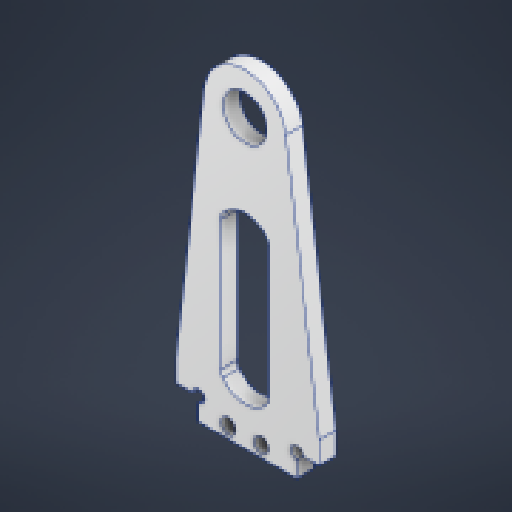
# Autodesk Inventor part: Leg_joint_slider_frame
Saved by Autodesk Inventor 2024 (Build 280153000, 153)
## iProperties
Created: 2024-01-23
Part Number: Leg_joint_slider_frame
Material: 알루미늄 6061
Document SubType Name: Modeling
Designer: ASUS
Density: 2.7 g/cm^3
Appearance: 알루미늄 - 평지
Mass: 6.96324 g
Surface Area: 24.9721 cm^2
Volume: 2.57898 cm^3
Author: ASUS
Autodesk Inventor part; units mm, degrees
ref_plane "YZ Plane" through (0, 0, 0) normal (1, 0, 0) x (0, 1, 0)
ref_plane "XZ Plane" through (0, 0, 0) normal (0, 1, 0) x (-1, 0, 0)
ref_plane "XY Plane" through (0, 0, 0) normal (0, 0, 1) x (1, 0, 0)
sketch "스케치1" plane through (0, 0, 0) normal (0, 0, 1) x (1, 0, 0)
  circle A0 centre (3, 0) radius 3 projected
  line L0 (7.4, -0.9434) -> (7.4, 0.9434) projected
  arc A1 (7.4, 0.9434) -> (-1.4, 0.9434) centre (3, 0) ccw projected
  line L1 (-1.4, 0.9434) -> (-1.4, -0.9434) projected
  arc A2 (-1.4, -0.9434) -> (7.4, -0.9434) centre (3, 0) ccw projected
  circle A3 centre (3, 20) radius 2.75 projected
  line L2 (3, 20) -> (3, 0)
  line L3 (3, 20) -> (3, 40)
  circle A4 centre (3, 40) radius 2.75
  circle A5 centre (3, 40) radius 7.5
  circle A6 centre (3, 0) radius 12.5
  line L4 (16.7123, -8.8378) -> (8.966, 52.6461)
  line L5 (-2.8681, 53.4235) -> (-11.5752, -15.6873)
  point P0 (0, 0)
  point P1 (10.4412, 40.9375)
  point P2 (-4.4412, 40.9375)
  point P3 (-9.402, 1.5625)
  point P4 (15.402, 1.5625)
  dimension "d2" = 360
  dimension "d4" = 5.5
  dimension "d5" = 15
  dimension "d6" = 25
  constraints: 8 end point, 5 coincident, 4 tangent, 3 centre point, 1 horizontal alignment, 1 vertical, 5 other
  measures "d4" diameter of A4
  measures "d5" diameter of A5
  measures "d6" diameter of A6
extrude "돌출1" add sketch "스케치1" along normal blind 3 contours A3 L3 A5 L4 A6 L2 | A3 L2 A6 L5 A5 L3 | A5 | A6
sketch "스케치2" plane through (0, 0, 3) normal (0, 0, 1) x (1, 0, 0)
  line L0 (-4.4412, 40.9375) -> (-9.402, 1.5625) projected
  arc A0 (-9.402, 1.5625) -> (15.402, 1.5625) centre (3, 0) ccw projected
  line L1 (15.402, 1.5625) -> (10.4412, 40.9375) projected
  arc A1 (10.4412, 40.9375) -> (-4.4412, 40.9375) centre (3, 40) ccw projected
  circle A2 centre (3, 40) radius 2.75 projected
  circle A3 centre (3, 20) radius 2.75 projected
  arc A4 (7.4, 0.9434) -> (-1.4, 0.9434) centre (3, 0) ccw projected
  line L2 (7.4, 0.9434) -> (7.4, -0.9434) projected
  arc A5 (-1.4, -0.9434) -> (7.4, -0.9434) centre (3, 0) ccw projected
  line L3 (-1.4, -0.9434) -> (-1.4, 0.9434) projected
  line L4 (-1.4, 14.3273) -> (-1.4, 9.5775) projected
  arc A6 (7.4, 14.3273) -> (-1.4, 14.3273) centre (3, 11.9524) ccw projected
  line L5 (7.4, 9.5775) -> (7.4, 14.3273) projected
  arc A7 (-1.4, 9.5775) -> (7.4, 9.5775) centre (3, 11.9524) ccw projected
  circle A8 centre (3, 11.9524) radius 6 projected
  line L6 (-1.4, 14.3273) -> (-1.4, -0.9434)
  line L7 (7.4, 14.3273) -> (7.4, -0.9434)
  point P0 (0, 0)
  point P1 (-1.4, 0.9434)
  point P2 (7.4, 0.9434)
  constraints: 4 end point, 1 parallel, 1 vertical
extrude "돌출2" cut sketch "스케치2" against normal up to surface (3 mm away) contours L6 A7 L7 A8 | A8 L7 A4 L6 | L4 A6 L5 A7
sketch "스케치3" plane through (0, 0, 0) normal (0, 0, -1) x (-1, 0, 0)
  circle A0 centre (-3, 40) radius 3.7 projected
  point P0 (0, 0)
extrude "돌출3" cut sketch "스케치3" against normal through all
sketch "스케치4" plane through (0, 0, 3) normal (0, 0, 1) x (1, 0, 0)
  circle A0 centre (3, 40) radius 4 projected
  circle A1 centre (3, 40) radius 3.7 projected
  line L0 (-1.4, -0.9434) -> (-1.4, 14.3273) projected
  arc A2 (7.4, 14.3273) -> (-1.4, 14.3273) centre (3, 11.9524) ccw projected
  line L1 (7.4, 14.3273) -> (7.4, -0.9434) projected
  arc A3 (-1.4, -0.9434) -> (7.4, -0.9434) centre (3, 0) ccw projected
  circle A4 centre (3, 20) radius 2.75 projected
  line L2 (-4.4412, 40.9375) -> (-9.402, 1.5625) projected
  arc A5 (-9.402, 1.5625) -> (15.402, 1.5625) centre (3, 0) ccw projected
  line L3 (15.402, 1.5625) -> (10.4412, 40.9375) projected
  arc A6 (10.4412, 40.9375) -> (-4.4412, 40.9375) centre (3, 40) ccw projected
  point P0 (0, 0)
extrude "돌출4" cut sketch "스케치4" against normal through all contours A0 | A1
sketch "스케치5" plane through (0, 0, 3) normal (0, 0, 1) x (1, 0, 0)
  circle A0 centre (3, 40) radius 4 projected
  line L0 (-1.4, -0.9434) -> (-1.4, 14.3273) projected
  arc A1 (7.4, 14.3273) -> (-1.4, 14.3273) centre (3, 11.9524) ccw projected
  line L1 (7.4, 14.3273) -> (7.4, -0.9434) projected
  arc A2 (-1.4, -0.9434) -> (7.4, -0.9434) centre (3, 0) ccw projected
  circle A3 centre (3, 20) radius 2.75 projected
  line L2 (-4.4412, 40.9375) -> (-9.402, 1.5625) projected
  arc A4 (-9.402, 1.5625) -> (15.402, 1.5625) centre (3, 0) ccw projected
  line L3 (15.402, 1.5625) -> (10.4412, 40.9375) projected
  arc A5 (10.4412, 40.9375) -> (-4.4412, 40.9375) centre (3, 40) ccw projected
  point P0 (0, 0)
extrude "돌출5" add sketch "스케치5" against normal up to surface (3 mm away) contours A3
sketch "스케치6" plane through (0, 0, 3) normal (0, 0, 1) x (1, 0, 0)
  circle A0 centre (3, 40) radius 4 projected
  line L0 (-1.4, -0.9434) -> (-1.4, 14.3273) projected
  arc A1 (7.4, 14.3273) -> (-1.4, 14.3273) centre (3, 11.9524) ccw projected
  line L1 (7.4, 14.3273) -> (7.4, -0.9434) projected
  arc A2 (-1.4, -0.9434) -> (7.4, -0.9434) centre (3, 0) ccw projected
  line L2 (-4.4412, 40.9375) -> (-9.402, 1.5625) projected
  arc A3 (-9.402, 1.5625) -> (15.402, 1.5625) centre (3, 0) ccw projected
  line L3 (15.402, 1.5625) -> (10.4412, 40.9375) projected
  arc A4 (10.4412, 40.9375) -> (-4.4412, 40.9375) centre (3, 40) ccw projected
  line L4 (-6.4255, 1.1875) -> (-1.4647, 40.5625)
  arc A5 (7.4647, 40.5625) -> (-1.4647, 40.5625) centre (3, 40) ccw
  line L5 (7.4647, 40.5625) -> (12.4255, 1.1875)
  arc A6 (-6.4255, 1.1875) -> (12.4255, 1.1875) centre (3, 0) ccw
  circle A7 centre (3, 40) radius 7
  circle A8 centre (3, 11.9524) radius 8.0059
  point P0 (0, 0)
  point P1 (-4.9432, 12.9531)
  point P2 (10.9432, 12.9531)
  point P3 (8.1349, 35.2427)
  point P4 (-2.1349, 35.2427)
  dimension "d17" = 3
  dimension "d18" = 3
  constraints: 4 centre point, 4 end point, 4 point on circle, 1 coincident, 1 tangent, 3 other
  measures "d17" distance between parallel lines of L2 L4
  measures "d18" radial gap between concentric circles of A0 A7
extrude "돌출6" cut sketch "스케치6" against normal through all contours L4 A7 L5 A8
fillet "모깎기1" radius 2 4 edges at (-2.1349, 35.2427, 1.5) (8.1349, 35.2427, 1.5) (-4.9432, 12.9531, 1.5) (10.9432, 12.9531, 1.5)
sketch "스케치8" plane through (0, 0, 3) normal (0, 0, 1) x (1, 0, 0)
  arc A0 (0.2302, 33.5713) -> (5.7698, 33.5713) centre (3, 40) ccw projected
  arc A1 (0.2302, 33.5713) -> (-2.5454, 31.9845) centre (-0.5611, 31.7345) ccw projected
  line L0 (-2.5454, 31.9845) -> (-3.9428, 20.8933) projected
  arc A2 (-3.9428, 20.8933) -> (-0.9674, 18.9062) centre (-1.9585, 20.6433) ccw projected
  arc A3 (6.9674, 18.9062) -> (-0.9674, 18.9062) centre (3, 11.9524) ccw projected
  arc A4 (6.9674, 18.9062) -> (9.9428, 20.8933) centre (7.9585, 20.6433) ccw projected
  line L1 (9.9428, 20.8933) -> (8.5454, 31.9845) projected
  arc A5 (8.5454, 31.9845) -> (5.7698, 33.5713) centre (6.5611, 31.7345) ccw projected
  circle A6 centre (3, 40) radius 4 projected
  line L2 (-1.4, 14.3273) -> (-1.4, -0.9434) projected
  arc A7 (-1.4, -0.9434) -> (7.4, -0.9434) centre (3, 0) ccw projected
  line L3 (7.4, -0.9434) -> (7.4, 14.3273) projected
  arc A8 (7.4, 14.3273) -> (-1.4, 14.3273) centre (3, 11.9524) ccw projected
  line L4 (-4.4412, 40.9375) -> (-9.402, 1.5625) projected
  arc A9 (10.4412, 40.9375) -> (-4.4412, 40.9375) centre (3, 40) ccw projected
  line L5 (15.402, 1.5625) -> (10.4412, 40.9375) projected
  arc A10 (-9.402, 1.5625) -> (15.402, 1.5625) centre (3, 0) ccw projected
  arc A11 (-1.4, 9.3409) -> (7.4, 9.3409) centre (3, 11.7157) ccw projected
  arc A12 (7.4, 14.0906) -> (-1.4, 14.0906) centre (3, 11.7157) ccw projected
  point P0 (0, 0)
extrude "돌출8" add sketch "스케치8" against normal up to surface (3 mm away) contours A8 L3 A12 L2
sketch "스케치9" plane through (0, 0, 0) normal (0, 0, -1) x (-1, 0, 0)
  line L0 (10.45, -12) -> (-15.45, -12)
  line L1 (10.45, -12) -> (10.45, -8)
  line L2 (-15.45, -8) -> (10.45, -8)
  line L3 (-15.45, -12) -> (-15.45, -8)
  arc A0 (-5.7698, 33.5713) -> (-0.2302, 33.5713) centre (-3, 40) ccw projected
  arc A1 (2.5454, 31.9845) -> (-0.2302, 33.5713) centre (0.5611, 31.7345) ccw projected
  line L4 (2.5454, 31.9845) -> (3.9428, 20.8933) projected
  arc A2 (0.9674, 18.9062) -> (3.9428, 20.8933) centre (1.9585, 20.6433) ccw projected
  arc A3 (0.9674, 18.9062) -> (-6.9674, 18.9062) centre (-3, 11.9524) ccw projected
  arc A4 (-9.9428, 20.8933) -> (-6.9674, 18.9062) centre (-7.9585, 20.6433) ccw projected
  line L5 (-9.9428, 20.8933) -> (-8.5454, 31.9845) projected
  arc A5 (-5.7698, 33.5713) -> (-8.5454, 31.9845) centre (-6.5611, 31.7345) ccw projected
  circle A6 centre (-3, 40) radius 4 projected
  line L6 (1.4, 14.0906) -> (1.4, -0.9434) projected
  arc A7 (-7.4, -0.9434) -> (1.4, -0.9434) centre (-3, 0) ccw projected
  line L7 (-7.4, -0.9434) -> (-7.4, 14.0906) projected
  arc A8 (1.4, 14.0906) -> (-7.4, 14.0906) centre (-3, 11.7157) ccw projected
  line L8 (4.4412, 40.9375) -> (9.402, 1.5625) projected
  arc A9 (4.4412, 40.9375) -> (-10.4412, 40.9375) centre (-3, 40) ccw projected
  line L9 (-15.402, 1.5625) -> (-10.4412, 40.9375) projected
  arc A10 (-15.402, 1.5625) -> (9.402, 1.5625) centre (-3, 0) ccw projected
  circle A11 centre (-3, 0) radius 12.5
  line L10 (-3, 0) -> (-15.5, 0)
  line L11 (-15.5, 0) -> (9.5, 0)
  line L12 (9.5, 0) -> (-15.5, 0)
  line L13 (-15.5, 0) -> (-15.5, -12)
  line L14 (-15.5, -12) -> (9.5, -12)
  line L15 (9.5, -12) -> (9.5, 0)
  point P0 (0, 0)
  point P1 (-6.5, -12)
  point P2 (0.5, -12)
  constraints: 20 end point, 3 equal length, 3 horizontal, 2 point on circle, 2 vertical, 1 centre point, 1 coincident, 1 perpendicular, 4 other
extrude "돌출9" add sketch "스케치9" against normal up to surface (3 mm away) contours L0 A10 L2 L15 | L2 A10 L15 | L0 L3 L2 A10 | L14 L13 A10 L2 L3
sketch "스케치10" plane through (0, 0, 0) normal (0, 0, -1) x (-1, 0, 0)
  arc A0 (-5.7698, 33.5713) -> (-0.2302, 33.5713) centre (-3, 40) ccw projected
  arc A1 (2.5454, 31.9845) -> (-0.2302, 33.5713) centre (0.5611, 31.7345) ccw projected
  line L0 (2.5454, 31.9845) -> (3.9428, 20.8933) projected
  arc A2 (0.9674, 18.9062) -> (3.9428, 20.8933) centre (1.9585, 20.6433) ccw projected
  arc A3 (0.9674, 18.9062) -> (-6.9674, 18.9062) centre (-3, 11.9524) ccw projected
  arc A4 (-9.9428, 20.8933) -> (-6.9674, 18.9062) centre (-7.9585, 20.6433) ccw projected
  line L1 (-9.9428, 20.8933) -> (-8.5454, 31.9845) projected
  arc A5 (-5.7698, 33.5713) -> (-8.5454, 31.9845) centre (-6.5611, 31.7345) ccw projected
  circle A6 centre (-3, 40) radius 4 projected
  line L2 (1.4, 14.0906) -> (1.4, -0.9434) projected
  arc A7 (-7.4, -0.9434) -> (1.4, -0.9434) centre (-3, 0) ccw projected
  line L3 (-7.4, -0.9434) -> (-7.4, 14.0906) projected
  arc A8 (1.4, 14.0906) -> (-7.4, 14.0906) centre (-3, 11.7157) ccw projected
  line L4 (4.4412, 40.9375) -> (9.402, 1.5625) projected
  arc A9 (4.4412, 40.9375) -> (-10.4412, 40.9375) centre (-3, 40) ccw projected
  line L5 (-15.402, 1.5625) -> (-10.4412, 40.9375) projected
  arc A10 (-15.402, 1.5625) -> (-15.5, 0) centre (-3, 0) ccw projected
  line L6 (-15.5, 0) -> (-15.5, -12) projected
  line L7 (-15.5, -12) -> (-6.5, -12) projected
  arc A11 (-6.5, -12) -> (0.5, -12) centre (-3, 0) ccw projected
  line L8 (0.5, -12) -> (9.5, -12) projected
  line L9 (9.5, -12) -> (9.5, 0) projected
  arc A12 (9.5, 0) -> (9.402, 1.5625) centre (-3, 0) ccw projected
  line L10 (9.5, -12) -> (-15.5, -12)
  point P0 (0, 0)
  constraints: 2 end point, 1 horizontal
extrude "돌출10" cut sketch "스케치10" against normal through all contours A11 L10
sketch "스케치11" plane through (0, 0, 0) normal (0, 0, -1) x (-1, 0, 0)
  line L0 (-8.5, -12) -> (3.5, -12)
  line L1 (-8.5, -8) -> (-8.5, -12)
  line L2 (3.5, -8) -> (-8.5, -8)
  line L3 (3.5, -12) -> (3.5, -8)
  line L4 (3.5, -10) -> (0.5, -10)
  line L5 (3.5, -10) -> (6.5, -10) construction
  line L6 (-8.5, -10) -> (-5.5, -10)
  line L7 (-8.5, -10) -> (-5.5, -10) construction
  circle A0 centre (0.5, -10) radius 1.35
  circle A1 centre (-5.5, -10) radius 1.35
  line L8 (-15.5, -12) -> (9.5, -12) projected
  line L9 (9.5, -12) -> (9.5, 0) projected
  arc A2 (9.5, 0) -> (9.402, 1.5625) centre (-3, 0) ccw projected
  line L10 (4.4412, 40.9375) -> (9.402, 1.5625) projected
  arc A3 (4.4412, 40.9375) -> (-10.4412, 40.9375) centre (-3, 40) ccw projected
  line L11 (-15.402, 1.5625) -> (-10.4412, 40.9375) projected
  arc A4 (-15.402, 1.5625) -> (-15.5, 0) centre (-3, 0) ccw projected
  line L12 (-15.5, 0) -> (-15.5, -12) projected
  line L13 (1.4, 14.0906) -> (1.4, -0.9434) projected
  arc A5 (-7.4, -0.9434) -> (1.4, -0.9434) centre (-3, 0) ccw projected
  line L14 (-7.4, -0.9434) -> (-7.4, 14.0906) projected
  arc A6 (1.4, 14.0906) -> (-7.4, 14.0906) centre (-3, 11.7157) ccw projected
  circle A7 centre (-3, 40) radius 4 projected
  arc A8 (-5.7698, 33.5713) -> (-0.2302, 33.5713) centre (-3, 40) ccw projected
  arc A9 (2.5454, 31.9845) -> (-0.2302, 33.5713) centre (0.5611, 31.7345) ccw projected
  line L15 (2.5454, 31.9845) -> (3.9428, 20.8933) projected
  arc A10 (0.9674, 18.9062) -> (3.9428, 20.8933) centre (1.9585, 20.6433) ccw projected
  arc A11 (0.9674, 18.9062) -> (-6.9674, 18.9062) centre (-3, 11.9524) ccw projected
  arc A12 (-9.9428, 20.8933) -> (-6.9674, 18.9062) centre (-7.9585, 20.6433) ccw projected
  line L16 (-9.9428, 20.8933) -> (-8.5454, 31.9845) projected
  arc A13 (-5.7698, 33.5713) -> (-8.5454, 31.9845) centre (-6.5611, 31.7345) ccw projected
  circle A14 centre (-3, 0) radius 13.6473
  line L17 (-3, 0) -> (-3, -10)
  line L18 (-5.5, -10) -> (0.5, -10)
  line L19 (9.896, -15.3181) -> (21.896, -15.3181)
  line L20 (9.896, -11.3181) -> (9.896, -15.3181)
  line L21 (21.896, -11.3181) -> (9.896, -11.3181)
  line L22 (21.896, -15.3181) -> (21.896, -11.3181)
  line L23 (21.896, -13.3181) -> (18.896, -13.3181)
  line L24 (9.896, -13.3181) -> (12.896, -13.3181)
  line L25 (9.896, -13.3181) -> (12.896, -13.3181) construction
  circle A15 centre (18.896, -13.3181) radius 1.35
  circle A16 centre (12.896, -13.3181) radius 1.35
  line L26 (12.896, -13.3181) -> (18.896, -13.3181)
  circle A17 centre (15.896, -13.3181) radius 0.4879
  line L27 (-9, -10) -> (-6, -10) construction
  line L28 (-9, -10) -> (-6, -10)
  line L29 (-9, -8) -> (-9, -12)
  circle A18 centre (-6, -10) radius 1.35
  line L30 (-6, -10) -> (0, -10)
  circle A19 centre (0, -10) radius 1.35
  line L31 (3, -10) -> (0, -10)
  line L32 (-9, -12) -> (3, -12)
  line L33 (3, -12) -> (3, -8)
  line L34 (3, -8) -> (-9, -8)
  circle A20 centre (-3, -10) radius 0.4879
  point P0 (0, 0)
  point P1 (-9.5, -12)
  point P2 (-15.5, -5.4772)
  point P3 (9.5, -5.4772)
  point P4 (15.396, -13.3181)
  point P5 (-3.5, -10)
  dimension "d30" = 3
  dimension "d31" = 180
  dimension "d32" = 3
  dimension "d33" = 0
  dimension "d34" = 2.7
  dimension "d35" = 2.7
  dimension "d44" = 3
  dimension "d45" = 3
  dimension "d46" = 0
  dimension "d47" = 2.7
  dimension "d48" = 2.7
  dimension "d49" = 3
  dimension "d50" = 3
  dimension "d51" = 0
  dimension "d52" = 2.7
  dimension "d53" = 2.7
  constraints: 52 end point, 19 horizontal, 8 centre point, 8 midpoint, 7 coincident, 7 vertical, 4 collinear, 15 other
  measures "d30" distance of L4.start L4.end
  measures "d31" angle of L4 L5
  measures "d32" distance of L6.start L6.end
  measures "d33" distance between parallel lines of L6 L7
  measures "d34" diameter of A0
  measures "d35" diameter of A1
  measures "d44" distance of L23.start L23.end
  measures "d45" distance of L25.start L24.end
  measures "d46" distance between parallel lines of L24 L25
  measures "d47" diameter of A15
  measures "d48" diameter of A16
  measures "d49" distance of L31.start L31.end
  measures "d50" distance of L28.start L28.end
  measures "d51" distance between parallel lines of L28 L27
  measures "d52" diameter of A19
  measures "d53" diameter of A18
extrude "돌출11" cut sketch "스케치11" against normal through all contours A18 A1 L6 | L6 A1 A18 | A1 A18 L18 L6 | L6 L18 A18 A1 | A19 A0 L18 L4 | L4 L18 A0 A19 | A0 L18 A19 | A19 L18 A0
sketch "스케치12" plane through (0, 0, 0) normal (0, 0, -1) x (-1, 0, 0)
  line L0 (-15.5, -12) -> (9.5, -12) projected
  line L1 (9.5, -12) -> (9.5, 0) projected
  arc A0 (9.5, 0) -> (9.402, 1.5625) centre (-3, 0) ccw projected
  line L2 (4.4412, 40.9375) -> (9.402, 1.5625) projected
  arc A1 (4.4412, 40.9375) -> (-10.4412, 40.9375) centre (-3, 40) ccw projected
  line L3 (-15.402, 1.5625) -> (-10.4412, 40.9375) projected
  arc A2 (-15.402, 1.5625) -> (-15.5, 0) centre (-3, 0) ccw projected
  line L4 (-15.5, 0) -> (-15.5, -12) projected
  line L5 (1.4, 14.0906) -> (1.4, -0.9434) projected
  arc A3 (-7.4, -0.9434) -> (1.4, -0.9434) centre (-3, 0) ccw projected
  line L6 (-7.4, -0.9434) -> (-7.4, 14.0906) projected
  arc A4 (1.4, 14.0906) -> (-7.4, 14.0906) centre (-3, 11.7157) ccw projected
  circle A5 centre (-3, 40) radius 4 projected
  arc A6 (-5.7698, 33.5713) -> (-0.2302, 33.5713) centre (-3, 40) ccw projected
  arc A7 (2.5454, 31.9845) -> (-0.2302, 33.5713) centre (0.5611, 31.7345) ccw projected
  line L7 (2.5454, 31.9845) -> (3.9428, 20.8933) projected
  arc A8 (0.9674, 18.9062) -> (3.9428, 20.8933) centre (1.9585, 20.6433) ccw projected
  arc A9 (0.9674, 18.9062) -> (-6.9674, 18.9062) centre (-3, 11.9524) ccw projected
  arc A10 (-9.9428, 20.8933) -> (-6.9674, 18.9062) centre (-7.9585, 20.6433) ccw projected
  line L8 (-9.9428, 20.8933) -> (-8.5454, 31.9845) projected
  arc A11 (-5.7698, 33.5713) -> (-8.5454, 31.9845) centre (-6.5611, 31.7345) ccw projected
  line L9 (9.5, -12) -> (-15.5, -12)
  line L10 (-15.5, -12) -> (-15.5, -13.5)
  line L11 (-15.5, -13.5) -> (9.5, -13.5)
  line L12 (9.5, -13.5) -> (9.5, -12)
  point P0 (0, 0)
  dimension "d38" = 1.5
  constraints: 8 end point, 3 equal length, 1 perpendicular
  measures "d38" distance of L10.end L0.start
extrude "돌출12" add sketch "스케치12" against normal up to surface (3 mm away) contours L0 L12 L11 L10
sketch "스케치13" plane through (0, 0, 0) normal (0, 0, -1) x (-1, 0, 0)
  line L0 (9.5, -13.5) -> (9.5, 0) projected
  arc A0 (9.5, 0) -> (9.402, 1.5625) centre (-3, 0) ccw projected
  line L1 (4.4412, 40.9375) -> (9.402, 1.5625) projected
  arc A1 (4.4412, 40.9375) -> (-10.4412, 40.9375) centre (-3, 40) ccw projected
  line L2 (-15.402, 1.5625) -> (-10.4412, 40.9375) projected
  arc A2 (-15.402, 1.5625) -> (-15.5, 0) centre (-3, 0) ccw projected
  line L3 (-15.5, 0) -> (-15.5, -13.5) projected
  line L4 (-15.5, -13.5) -> (9.5, -13.5) projected
  line L5 (1.4, 14.0906) -> (1.4, -0.9434) projected
  arc A3 (-7.4, -0.9434) -> (1.4, -0.9434) centre (-3, 0) ccw projected
  line L6 (-7.4, -0.9434) -> (-7.4, 14.0906) projected
  arc A4 (1.4, 14.0906) -> (-7.4, 14.0906) centre (-3, 11.7157) ccw projected
  circle A5 centre (-3, 40) radius 4 projected
  arc A6 (-5.7698, 33.5713) -> (-0.2302, 33.5713) centre (-3, 40) ccw projected
  arc A7 (2.5454, 31.9845) -> (-0.2302, 33.5713) centre (0.5611, 31.7345) ccw projected
  line L7 (2.5454, 31.9845) -> (3.9428, 20.8933) projected
  arc A8 (0.9674, 18.9062) -> (3.9428, 20.8933) centre (1.9585, 20.6433) ccw projected
  arc A9 (0.9674, 18.9062) -> (-6.9674, 18.9062) centre (-3, 11.9524) ccw projected
  arc A10 (-9.9428, 20.8933) -> (-6.9674, 18.9062) centre (-7.9585, 20.6433) ccw projected
  line L8 (-9.9428, 20.8933) -> (-8.5454, 31.9845) projected
  arc A11 (-5.7698, 33.5713) -> (-8.5454, 31.9845) centre (-6.5611, 31.7345) ccw projected
  circle A12 centre (-3, 0) radius 13.5
  point P0 (0, 0)
  point P1 (-3, -13.5)
  point P2 (-15.5, -5.099)
  point P3 (9.5, -5.099)
  constraints: 1 centre point, 1 coincident, 1 tangent
extrude "돌출13" cut sketch "스케치13" against normal through all contours L4 A12 L0 | L4 L3 A12
fillet "모깎기2" radius 10 2 edges at (-9.5, -5.099, 1.5) (15.5, -5.099, 1.5)
sketch "스케치14" plane through (0, 0, 3) normal (0, 0, 1) x (1, 0, 0)
  line L0 (7.4, -2.3749) -> (7.4, 2.3749)
  arc A0 (7.4, 2.3749) -> (-1.4, 2.3749) centre (3, 0) ccw
  arc A1 (12.6429, -9.448) -> (15.5, -2.4495) centre (5.5, -2.4495) ccw projected
  line L1 (15.5, 0) -> (15.5, -2.4495) projected
  arc A2 (15.5, 0) -> (15.402, 1.5625) centre (3, 0) ccw projected
  line L2 (15.402, 1.5625) -> (10.4412, 40.9375) projected
  arc A3 (10.4412, 40.9375) -> (-4.4412, 40.9375) centre (3, 40) ccw projected
  line L3 (-4.4412, 40.9375) -> (-9.402, 1.5625) projected
  arc A4 (-9.402, 1.5625) -> (-9.5, 0) centre (3, 0) ccw projected
  line L4 (-9.5, -2.4495) -> (-9.5, 0) projected
  arc A5 (-9.5, -2.4495) -> (-6.6429, -9.448) centre (0.5, -2.4495) ccw projected
  arc A6 (-6.6429, -9.448) -> (12.6429, -9.448) centre (3, 0) ccw projected
  circle A7 centre (6, -10) radius 1.35 projected
  circle A8 centre (0, -10) radius 1.35 projected
  arc A9 (0.2302, 33.5713) -> (5.7698, 33.5713) centre (3, 40) ccw projected
  arc A10 (8.5454, 31.9845) -> (5.7698, 33.5713) centre (6.5611, 31.7345) ccw projected
  line L5 (8.5454, 31.9845) -> (9.9428, 20.8933) projected
  arc A11 (6.9674, 18.9062) -> (9.9428, 20.8933) centre (7.9585, 20.6433) ccw projected
  arc A12 (6.9674, 18.9062) -> (-0.9674, 18.9062) centre (3, 11.9524) ccw projected
  arc A13 (-3.9428, 20.8933) -> (-0.9674, 18.9062) centre (-1.9585, 20.6433) ccw projected
  line L6 (-3.9428, 20.8933) -> (-2.5454, 31.9845) projected
  arc A14 (0.2302, 33.5713) -> (-2.5454, 31.9845) centre (-0.5611, 31.7345) ccw projected
  circle A15 centre (3, 40) radius 4 projected
  line L7 (-1.4, -0.9434) -> (-1.4, 14.0906) projected
  arc A16 (7.4, 14.0906) -> (-1.4, 14.0906) centre (3, 11.7157) ccw projected
  line L8 (7.4, 14.0906) -> (7.4, -0.9434) projected
  arc A17 (-1.4, -0.9434) -> (7.4, -0.9434) centre (3, 0) ccw projected
  arc A18 (-1.4, -2.3749) -> (7.4, -2.3749) centre (3, 0) ccw
  line L9 (-1.4, 2.3749) -> (-1.4, -2.3749)
  point P0 (0, 0)
  constraints: 4 end point, 4 point on circle, 2 centre point, 2 vertical, 8 other
extrude "돌출14" cut sketch "스케치14" against normal through all contours A18 L9 A17 L0
sketch "스케치15" plane through (0, 0, 3) normal (0, 0, 1) x (1, 0, 0)
  circle A0 centre (3, 11.7157) radius 6
  line L0 (7.4, 12.6591) -> (7.4, 10.7723)
  arc A1 (7.4, 12.6591) -> (-1.4, 12.6591) centre (3, 11.7157) ccw
  arc A2 (-1.4, 10.7723) -> (7.4, 10.7723) centre (3, 11.7157) ccw
  line L1 (-1.4, -2.3749) -> (-1.4, 14.0906) projected
  arc A3 (7.4, 14.0906) -> (-1.4, 14.0906) centre (3, 11.7157) ccw projected
  line L2 (7.4, 14.0906) -> (7.4, -2.3749) projected
  arc A4 (-1.4, -2.3749) -> (7.4, -2.3749) centre (3, 0) ccw projected
  arc A5 (12.6429, -9.448) -> (15.5, -2.4495) centre (5.5, -2.4495) ccw projected
  line L3 (15.5, 0) -> (15.5, -2.4495) projected
  arc A6 (15.5, 0) -> (15.402, 1.5625) centre (3, 0) ccw projected
  line L4 (15.402, 1.5625) -> (10.4412, 40.9375) projected
  arc A7 (10.4412, 40.9375) -> (-4.4412, 40.9375) centre (3, 40) ccw projected
  line L5 (-4.4412, 40.9375) -> (-9.402, 1.5625) projected
  arc A8 (-9.402, 1.5625) -> (-9.5, 0) centre (3, 0) ccw projected
  line L6 (-9.5, -2.4495) -> (-9.5, 0) projected
  arc A9 (-9.5, -2.4495) -> (-6.6429, -9.448) centre (0.5, -2.4495) ccw projected
  arc A10 (-6.6429, -9.448) -> (12.6429, -9.448) centre (3, 0) ccw projected
  circle A11 centre (6, -10) radius 1.35 projected
  circle A12 centre (0, -10) radius 1.35 projected
  arc A13 (0.2302, 33.5713) -> (5.7698, 33.5713) centre (3, 40) ccw projected
  arc A14 (8.5454, 31.9845) -> (5.7698, 33.5713) centre (6.5611, 31.7345) ccw projected
  line L7 (8.5454, 31.9845) -> (9.9428, 20.8933) projected
  arc A15 (6.9674, 18.9062) -> (9.9428, 20.8933) centre (7.9585, 20.6433) ccw projected
  arc A16 (6.9674, 18.9062) -> (-0.9674, 18.9062) centre (3, 11.9524) ccw projected
  arc A17 (-3.9428, 20.8933) -> (-0.9674, 18.9062) centre (-1.9585, 20.6433) ccw projected
  line L8 (-3.9428, 20.8933) -> (-2.5454, 31.9845) projected
  arc A18 (0.2302, 33.5713) -> (-2.5454, 31.9845) centre (-0.5611, 31.7345) ccw projected
  circle A19 centre (3, 40) radius 4 projected
  point P0 (0, 0)
  point P1 (-1.4, 12.6591)
  point P2 (7.4, 12.6591)
  constraints: 4 point on circle, 3 centre point, 2 end point, 1 vertical, 10 other
extrude "돌출15" add sketch "스케치15" against normal up to surface (3 mm away) contours L1 A3 L2 A1
sketch "스케치16" plane through (0, 0, 0) normal (0, 0, -1) x (-1, 0, 0)
  arc A0 (-7.398, 14.0944) -> (-2.5749, 6.7338) centre (-3, 11.7157) ccw
  circle A1 centre (-3, 11.7157) radius 5
  arc A2 (-7.4, -2.3749) -> (1.4, -2.3749) centre (-3, 0) ccw projected
  line L0 (-7.4, -2.3749) -> (1.4, -2.3749)
  line L1 (1.4, -2.3749) -> (1.4, 16.7157)
  line L2 (1.4, 16.7157) -> (-7.4, 16.7157)
  line L3 (-7.4, 16.7157) -> (-7.4, -2.3749)
  point P0 (0, 0)
  point P1 (1.4, 14.0906)
  point P2 (-7.398, 14.0944)
  point P3 (-7.4, 14.0906)
  constraints: 8 end point, 2 parallel, 2 point on circle, 1 centre point, 1 coincident, 1 horizontal, 1 perpendicular, 7 other
extrude "돌출16" cut sketch "스케치16" against normal through all contours A1 L1 A0 L3 | A0 A1 L1 L0 L3 | L0 A2
sketch "스케치17" plane through (0, 0, 0) normal (0, 0, -1) x (-1, 0, 0)
  arc A0 (-15.5, -2.4495) -> (-12.6429, -9.448) centre (-5.5, -2.4495) ccw projected
  arc A1 (-12.6429, -9.448) -> (6.6429, -9.448) centre (-3, 0) ccw projected
  arc A2 (6.6429, -9.448) -> (9.5, -2.4495) centre (-0.5, -2.4495) ccw projected
  line L0 (9.5, -2.4495) -> (9.5, 0) projected
  arc A3 (9.5, 0) -> (9.402, 1.5625) centre (-3, 0) ccw projected
  line L1 (4.4412, 40.9375) -> (9.402, 1.5625) projected
  arc A4 (4.4412, 40.9375) -> (-10.4412, 40.9375) centre (-3, 40) ccw projected
  line L2 (-15.402, 1.5625) -> (-10.4412, 40.9375) projected
  arc A5 (-15.402, 1.5625) -> (-15.5, 0) centre (-3, 0) ccw projected
  line L3 (-15.5, 0) -> (-15.5, -2.4495) projected
  arc A6 (-5.7698, 33.5713) -> (-0.2302, 33.5713) centre (-3, 40) ccw projected
  arc A7 (2.5454, 31.9845) -> (-0.2302, 33.5713) centre (0.5611, 31.7345) ccw projected
  line L4 (2.5454, 31.9845) -> (3.9428, 20.8933) projected
  arc A8 (0.9674, 18.9062) -> (3.9428, 20.8933) centre (1.9585, 20.6433) ccw projected
  arc A9 (0.9674, 18.9062) -> (-6.9674, 18.9062) centre (-3, 11.9524) ccw projected
  arc A10 (-9.9428, 20.8933) -> (-6.9674, 18.9062) centre (-7.9585, 20.6433) ccw projected
  line L5 (-9.9428, 20.8933) -> (-8.5454, 31.9845) projected
  arc A11 (-5.7698, 33.5713) -> (-8.5454, 31.9845) centre (-6.5611, 31.7345) ccw projected
  circle A12 centre (-3, 40) radius 4 projected
  line L6 (-7.4, -2.3749) -> (-7.4, 14.0906) projected
  arc A13 (1.4, 14.0906) -> (-7.4, 14.0906) centre (-3, 11.7157) ccw projected
  line L7 (1.4, 14.0906) -> (1.4, -2.3749) projected
  arc A14 (-7.4, -2.3749) -> (1.4, -2.3749) centre (-3, 0) ccw projected
  circle A15 centre (0, -10) radius 1.35 projected
  circle A16 centre (-6, -10) radius 1.35 projected
  line L8 (-6.4, 13.8229) -> (-6.4, -2.1071)
  arc A17 (-6.4, -2.1071) -> (0.4, -2.1071) centre (-3, 0) ccw
  line L9 (0.4, -2.1071) -> (0.4, 13.8229)
  arc A18 (0.4, 13.8229) -> (-6.4, 13.8229) centre (-3, 11.7157) ccw
  circle A19 centre (-6.4, 13.8229) radius 1.05
  circle A20 centre (0.4, 13.8229) radius 1.05
  circle A21 centre (-6.4, -2.1071) radius 1.05
  circle A22 centre (0.4, -2.1071) radius 1.05
  point P0 (0, 0)
  dimension "d60" = 1
  dimension "d61" = 2.1
  dimension "d62" = 2.1
  dimension "d63" = 2.1
  dimension "d64" = 2.1
  constraints: 6 centre point, 4 coincident, 4 end point, 4 point on circle, 3 other
  measures "d60" radial gap between concentric circles of A13 A18
  measures "d61" diameter of A19
  measures "d62" diameter of A20
  measures "d63" diameter of A21
  measures "d64" diameter of A22
extrude "돌출17" cut sketch "스케치17" against normal through all contours A14 A21 L6 | L6 A21 L8 A17 A14 | A19 A13 L6 | L6 A13 A19 A18 L8 | A21 A17 L8 | A22 A17 L9 L7 A14 | A14 L7 A22 | L8 A18 A19 | A22 L9 A17 | A20 L7 A13 | A13 L7 A20 L9 A18 | A18 L9 A20
sketch "스케치18" plane through (0, 0, 0) normal (0, 0, -1) x (-1, 0, 0)
  circle A0 centre (-6, -10) radius 1.35 projected
  circle A1 centre (0, -10) radius 1.35 projected
  circle A2 centre (-3, 40) radius 4 projected
  arc A3 (-5.7698, 33.5713) -> (-0.2302, 33.5713) centre (-3, 40) ccw projected
  arc A4 (2.5454, 31.9845) -> (-0.2302, 33.5713) centre (0.5611, 31.7345) ccw projected
  line L0 (2.5454, 31.9845) -> (3.9428, 20.8933) projected
  arc A5 (0.9674, 18.9062) -> (3.9428, 20.8933) centre (1.9585, 20.6433) ccw projected
  arc A6 (0.9674, 18.9062) -> (-6.9674, 18.9062) centre (-3, 11.9524) ccw projected
  arc A7 (-9.9428, 20.8933) -> (-6.9674, 18.9062) centre (-7.9585, 20.6433) ccw projected
  line L1 (-9.9428, 20.8933) -> (-8.5454, 31.9845) projected
  arc A8 (-5.7698, 33.5713) -> (-8.5454, 31.9845) centre (-6.5611, 31.7345) ccw projected
  arc A9 (-15.5, -2.4495) -> (-12.6429, -9.448) centre (-5.5, -2.4495) ccw projected
  arc A10 (-12.6429, -9.448) -> (6.6429, -9.448) centre (-3, 0) ccw projected
  arc A11 (6.6429, -9.448) -> (9.5, -2.4495) centre (-0.5, -2.4495) ccw projected
  line L2 (9.5, -2.4495) -> (9.5, 0) projected
  arc A12 (9.5, 0) -> (9.402, 1.5625) centre (-3, 0) ccw projected
  line L3 (4.4412, 40.9375) -> (9.402, 1.5625) projected
  arc A13 (4.4412, 40.9375) -> (-10.4412, 40.9375) centre (-3, 40) ccw projected
  line L4 (-15.402, 1.5625) -> (-10.4412, 40.9375) projected
  arc A14 (-15.402, 1.5625) -> (-15.5, 0) centre (-3, 0) ccw projected
  line L5 (-15.5, 0) -> (-15.5, -2.4495) projected
  arc A15 (-7.0507, 14.647) -> (-7.4, 13.5027) centre (-6.4, 13.8229) ccw projected
  arc A16 (1.0507, 14.647) -> (-7.0507, 14.647) centre (-3, 11.7157) ccw projected
  arc A17 (1.4, 13.5027) -> (1.0507, 14.647) centre (0.4, 13.8229) ccw projected
  line L6 (1.4, 13.5027) -> (1.4, -1.787) projected
  arc A18 (1.0507, -2.9312) -> (1.4, -1.787) centre (0.4, -2.1071) ccw projected
  arc A19 (-7.0507, -2.9312) -> (1.0507, -2.9312) centre (-3, 0) ccw projected
  arc A20 (-7.4, -1.787) -> (-7.0507, -2.9312) centre (-6.4, -2.1071) ccw projected
  line L7 (-7.4, -1.787) -> (-7.4, 13.5027) projected
  point P0 (0, 0)
extrude "돌출18" add sketch "스케치18" against normal blind 3 contours A3 A4 L0 A5 A6 A7 L1 A8
sketch "스케치19" plane through (0, 0, 0) normal (0, 0, -1) x (-1, 0, 0)
  circle A0 centre (-6, -10) radius 1.35 projected
  circle A1 centre (0, -10) radius 1.35 projected
  circle A2 centre (-3, 40) radius 4 projected
  arc A3 (-15.5, -2.4495) -> (-12.6429, -9.448) centre (-5.5, -2.4495) ccw projected
  arc A4 (-12.6429, -9.448) -> (6.6429, -9.448) centre (-3, 0) ccw projected
  arc A5 (6.6429, -9.448) -> (9.5, -2.4495) centre (-0.5, -2.4495) ccw projected
  line L0 (9.5, -2.4495) -> (9.5, 0) projected
  arc A6 (9.5, 0) -> (9.402, 1.5625) centre (-3, 0) ccw projected
  line L1 (4.4412, 40.9375) -> (9.402, 1.5625) projected
  arc A7 (4.4412, 40.9375) -> (-10.4412, 40.9375) centre (-3, 40) ccw projected
  line L2 (-15.402, 1.5625) -> (-10.4412, 40.9375) projected
  arc A8 (-15.402, 1.5625) -> (-15.5, 0) centre (-3, 0) ccw projected
  line L3 (-15.5, 0) -> (-15.5, -2.4495) projected
  arc A9 (-7.0507, 14.647) -> (-7.4, 13.5027) centre (-6.4, 13.8229) ccw projected
  arc A10 (1.0507, 14.647) -> (-7.0507, 14.647) centre (-3, 11.7157) ccw projected
  arc A11 (1.4, 13.5027) -> (1.0507, 14.647) centre (0.4, 13.8229) ccw projected
  line L4 (1.4, 13.5027) -> (1.4, -1.787) projected
  arc A12 (1.0507, -2.9312) -> (1.4, -1.787) centre (0.4, -2.1071) ccw projected
  arc A13 (-7.0507, -2.9312) -> (1.0507, -2.9312) centre (-3, 0) ccw projected
  arc A14 (-7.4, -1.787) -> (-7.0507, -2.9312) centre (-6.4, -2.1071) ccw projected
  line L5 (-7.4, -1.787) -> (-7.4, 13.5027) projected
  circle A15 centre (-3, 0) radius 5
  circle A16 centre (-3, 11.7157) radius 5
  line L6 (-3, 0) -> (-3, 20)
  line L7 (-3, 0) -> (17, 0) construction
  line L8 (-7.4, 13.5027) -> (1.4, 13.5027)
  line L9 (1.4, 13.5027) -> (1.4, 36)
  line L10 (1.4, 36) -> (-7.4, 36)
  line L11 (-7.4, 36) -> (-7.4, 13.5027)
  circle A17 centre (-3, 20) radius 5
  point P0 (0, 0)
  point P1 (-7.4, 14.143)
  point P2 (1.4, 14.143)
  point P3 (1.4, 22.3749)
  point P4 (-7.4, 22.3749)
  dimension "d69" = 20
  dimension "d70" = 90
  dimension "d71" = 10
  constraints: 12 end point, 3 centre point, 3 coincident, 3 perpendicular, 2 concentric, 2 parallel, 1 horizontal, 1 vertical
  measures "d69" distance of L6.start L6.end
  measures "d70" angle of L7 L6
  measures "d71" diameter of A17
extrude "돌출19" cut sketch "스케치19" against normal blind 3 contours L9 A17 A10 L11 | L9 A11 A10 A17 | A17 A10 A9 L11
sketch "스케치20" plane through (0, 0, 0) normal (0, 0, -1) x (-1, 0, 0)
  line L0 (1.4, 22.3749) -> (1.4, 14.143) projected
  arc A0 (1.4, 13.5027) -> (1.4, 14.143) centre (0.4, 13.8229) ccw projected
  line L1 (1.4, 13.5027) -> (1.4, -1.787) projected
  arc A1 (1.0507, -2.9312) -> (1.4, -1.787) centre (0.4, -2.1071) ccw projected
  arc A2 (-7.0507, -2.9312) -> (1.0507, -2.9312) centre (-3, 0) ccw projected
  arc A3 (-7.4, -1.787) -> (-7.0507, -2.9312) centre (-6.4, -2.1071) ccw projected
  line L2 (-7.4, -1.787) -> (-7.4, 13.5027) projected
  arc A4 (-7.4, 14.143) -> (-7.4, 13.5027) centre (-6.4, 13.8229) ccw projected
  line L3 (-7.4, 14.143) -> (-7.4, 22.3749) projected
  arc A5 (1.4, 22.3749) -> (-7.4, 22.3749) centre (-3, 20) ccw projected
  circle A6 centre (-6, -10) radius 1.35 projected
  circle A7 centre (0, -10) radius 1.35 projected
  circle A8 centre (-3, 40) radius 4 projected
  arc A9 (-15.5, -2.4495) -> (-12.6429, -9.448) centre (-5.5, -2.4495) ccw projected
  arc A10 (-12.6429, -9.448) -> (6.6429, -9.448) centre (-3, 0) ccw projected
  arc A11 (6.6429, -9.448) -> (9.5, -2.4495) centre (-0.5, -2.4495) ccw projected
  line L4 (9.5, -2.4495) -> (9.5, 0) projected
  arc A12 (9.5, 0) -> (9.402, 1.5625) centre (-3, 0) ccw projected
  line L5 (4.4412, 40.9375) -> (9.402, 1.5625) projected
  arc A13 (4.4412, 40.9375) -> (-10.4412, 40.9375) centre (-3, 40) ccw projected
  line L6 (-15.402, 1.5625) -> (-10.4412, 40.9375) projected
  arc A14 (-15.402, 1.5625) -> (-15.5, 0) centre (-3, 0) ccw projected
  line L7 (-15.5, 0) -> (-15.5, -2.4495) projected
  line L8 (-7.4, 22.3749) -> (1.4, 22.3749)
  line L9 (1.4, 22.3749) -> (1.4, -7.9312)
  line L10 (1.4, -7.9312) -> (-7.4, -7.9312)
  line L11 (-7.4, -7.9312) -> (-7.4, 22.3749)
  point P0 (0, 0)
  point P1 (1.4, 13.5027)
  point P2 (-7.4, 14.143)
  constraints: 8 end point, 2 parallel, 2 perpendicular
extrude "돌출20" add sketch "스케치20" against normal blind 3 contours A0 L9 | L11 A4
sketch "스케치21" plane through (0, 0, 0) normal (0, 0, -1) x (-1, 0, 0)
  line L0 (1.4, 22.3749) -> (1.4, -1.787) projected
  arc A0 (1.0507, -2.9312) -> (1.4, -1.787) centre (0.4, -2.1071) ccw projected
  arc A1 (-7.0507, -2.9312) -> (1.0507, -2.9312) centre (-3, 0) ccw projected
  arc A2 (-7.4, -1.787) -> (-7.0507, -2.9312) centre (-6.4, -2.1071) ccw projected
  line L1 (-7.4, -1.787) -> (-7.4, 22.3749) projected
  arc A3 (1.4, 22.3749) -> (-7.4, 22.3749) centre (-3, 20) ccw projected
  circle A4 centre (-6, -10) radius 1.35 projected
  circle A5 centre (0, -10) radius 1.35 projected
  circle A6 centre (-3, 40) radius 4 projected
  arc A7 (-15.5, -2.4495) -> (-12.6429, -9.448) centre (-5.5, -2.4495) ccw projected
  arc A8 (-12.6429, -9.448) -> (6.6429, -9.448) centre (-3, 0) ccw projected
  arc A9 (6.6429, -9.448) -> (9.5, -2.4495) centre (-0.5, -2.4495) ccw projected
  line L2 (9.5, -2.4495) -> (9.5, 0) projected
  arc A10 (9.5, 0) -> (9.402, 1.5625) centre (-3, 0) ccw projected
  line L3 (4.4412, 40.9375) -> (9.402, 1.5625) projected
  arc A11 (4.4412, 40.9375) -> (-10.4412, 40.9375) centre (-3, 40) ccw projected
  line L4 (-15.402, 1.5625) -> (-10.4412, 40.9375) projected
  arc A12 (-15.402, 1.5625) -> (-15.5, 0) centre (-3, 0) ccw projected
  line L5 (-15.5, 0) -> (-15.5, -2.4495) projected
  line L6 (-6.4, -2.1071) -> (-3, 0)
  line L7 (-3, 0) -> (0.4, -2.1071)
  line L8 (0.4, 27.1071) -> (-3, 25)
  line L9 (-3, 25) -> (-6.4, 27.1071)
  circle A13 centre (-6.4, 27.1071) radius 1.05
  circle A14 centre (0.4, 27.1071) radius 1.05
  line L10 (0.4, 22.1071) -> (-3, 20)
  line L11 (-3, 20) -> (-6.4, 22.1071)
  circle A15 centre (-6.4, 22.1071) radius 1.05
  circle A16 centre (0.4, 22.1071) radius 1.05
  point P0 (0, 0)
  point P1 (-3, 25)
  point P2 (-3, 20)
  dimension "d76" = 2.1
  dimension "d77" = 2.1
  dimension "d80" = 2.1
  dimension "d81" = 2.1
  constraints: 12 end point, 4 centre point, 4 coincident
  measures "d76" diameter of A13
  measures "d77" diameter of A14
  measures "d80" diameter of A15
  measures "d81" diameter of A16
extrude "돌출21" cut sketch "스케치21" against normal blind 3 contours A3 A16 L0 | L0 A16 A3 | A15 L1 A3 | A3 L1 A15
sketch "스케치22" plane through (0, 0, 3) normal (0, 0, 1) x (1, 0, 0)
  arc A0 (-1.0507, 22.9312) -> (-1.4, 21.787) centre (-0.4, 22.1071) ccw projected
  arc A1 (7.0507, 22.9312) -> (-1.0507, 22.9312) centre (3, 20) ccw projected
  arc A2 (7.4, 21.787) -> (7.0507, 22.9312) centre (6.4, 22.1071) ccw projected
  line L0 (7.4, 21.787) -> (7.4, -1.787) projected
  arc A3 (7.0507, -2.9312) -> (7.4, -1.787) centre (6.4, -2.1071) ccw projected
  arc A4 (-1.0507, -2.9312) -> (7.0507, -2.9312) centre (3, 0) ccw projected
  arc A5 (-1.4, -1.787) -> (-1.0507, -2.9312) centre (-0.4, -2.1071) ccw projected
  line L1 (-1.4, -1.787) -> (-1.4, 21.787) projected
  circle A6 centre (3, 40) radius 4 projected
  circle A7 centre (0, -10) radius 1.35 projected
  circle A8 centre (6, -10) radius 1.35 projected
  arc A9 (12.6429, -9.448) -> (15.5, -2.4495) centre (5.5, -2.4495) ccw projected
  line L2 (15.5, 0) -> (15.5, -2.4495) projected
  arc A10 (15.5, 0) -> (15.402, 1.5625) centre (3, 0) ccw projected
  line L3 (15.402, 1.5625) -> (10.4412, 40.9375) projected
  arc A11 (10.4412, 40.9375) -> (-4.4412, 40.9375) centre (3, 40) ccw projected
  line L4 (-4.4412, 40.9375) -> (-9.402, 1.5625) projected
  arc A12 (-9.402, 1.5625) -> (-9.5, 0) centre (3, 0) ccw projected
  line L5 (-9.5, -2.4495) -> (-9.5, 0) projected
  arc A13 (-9.5, -2.4495) -> (-6.6429, -9.448) centre (0.5, -2.4495) ccw projected
  arc A14 (-6.6429, -9.448) -> (12.6429, -9.448) centre (3, 0) ccw projected
  circle A15 centre (6, -10) radius 1.35 projected
  circle A16 centre (0, -10) radius 1.35 projected
  line L6 (16.45, -8) -> (-9.45, -8) projected
  line L7 (-9.45, -12) -> (-9.45, -8) projected
  line L8 (16.45, -12) -> (-9.45, -12) projected
  line L9 (16.45, -12) -> (16.45, -8) projected
  line L10 (-9.45, -12) -> (-9.45, 9.2219)
  line L11 (-9.45, -12) -> (11.7719, -12) construction
  line L12 (-9.45, 9.2219) -> (16.45, 9.2219)
  line L13 (16.45, 9.2219) -> (16.45, -12)
  line L14 (16.45, -12) -> (-9.45, -12)
  line L15 (-9.45, -12) -> (-9.45, 9.2219)
  line L16 (15.402, 1.5625) -> (10.4412, 40.9375) projected
  line L17 (15.402, 1.5625) -> (17.4518, -14.7074)
  point P0 (0, 0)
  point P1 (16.45, -6.7561)
  point P2 (9.1847, -12)
  point P3 (-3.1847, -12)
  point P4 (-9.45, -3.4482)
  dimension "d82" = 90
  constraints: 14 end point, 2 horizontal, 2 parallel, 2 perpendicular, 1 collinear
  measures "d82" angle of L11 L10
extrude "돌출22" add sketch "스케치22" against normal blind 3 contours L17 L13 L6 A9 L2 A10 | A13 L6 L10 | A13 A14 L8 L7 L6 | L9 L8 A14 A9 L6
sketch "스케치23" plane through (0, 0, 3) normal (0, 0, 1) x (1, 0, 0)
  arc A0 (-1.0507, 22.9312) -> (-1.4, 21.787) centre (-0.4, 22.1071) ccw projected
  arc A1 (7.0507, 22.9312) -> (-1.0507, 22.9312) centre (3, 20) ccw projected
  arc A2 (7.4, 21.787) -> (7.0507, 22.9312) centre (6.4, 22.1071) ccw projected
  line L0 (7.4, 21.787) -> (7.4, -1.787) projected
  arc A3 (7.0507, -2.9312) -> (7.4, -1.787) centre (6.4, -2.1071) ccw projected
  arc A4 (-1.0507, -2.9312) -> (7.0507, -2.9312) centre (3, 0) ccw projected
  arc A5 (-1.4, -1.787) -> (-1.0507, -2.9312) centre (-0.4, -2.1071) ccw projected
  line L1 (-1.4, -1.787) -> (-1.4, 21.787) projected
  circle A6 centre (3, 40) radius 4 projected
  circle A7 centre (0, -10) radius 1.35 projected
  circle A8 centre (6, -10) radius 1.35 projected
  line L2 (9.1847, -12) -> (16.45, -12) projected
  line L3 (16.45, -12) -> (16.45, -6.7561) projected
  line L4 (16.45, -6.7561) -> (10.4412, 40.9375) projected
  arc A9 (10.4412, 40.9375) -> (-4.4412, 40.9375) centre (3, 40) ccw projected
  line L5 (-4.4412, 40.9375) -> (-9.402, 1.5625) projected
  arc A10 (-9.402, 1.5625) -> (-9.5, 0) centre (3, 0) ccw projected
  line L6 (-9.5, -2.4495) -> (-9.5, 0) projected
  arc A11 (-9.5, -2.4495) -> (-9.45, -3.4482) centre (0.5, -2.4495) ccw projected
  line L7 (-9.45, -3.4482) -> (-9.45, -12) projected
  line L8 (-9.45, -12) -> (-3.1847, -12) projected
  arc A12 (-3.1847, -12) -> (9.1847, -12) centre (3, 0) ccw projected
  line L9 (-9.45, -12) -> (16.45, -12)
  line L10 (16.45, -12) -> (16.45, 19.622)
  line L11 (16.45, 19.622) -> (-9.45, 19.622)
  line L12 (-9.45, 19.622) -> (-9.45, -12)
  point P0 (0, 0)
  point P1 (-9.45, -3.4482)
  point P2 (-9.45, 1.1169)
  point P3 (-7.1267, 19.622)
  point P4 (13.1267, 19.622)
  constraints: 8 end point, 2 parallel, 1 collinear, 1 perpendicular
extrude "돌출23" cut sketch "스케치23" against normal through all contours L5 A10 L12 L11 | L11 L10 L4 | L12 A11 L6 A10 | A12 L9
sketch "스케치24" plane through (0, 0, 0) normal (0, 0, -1) x (-1, 0, 0)
  line L0 (9.45, -12) -> (-16.45, -12) projected
  line L1 (-16.45, -12) -> (9.45, -12) projected
  arc A0 (1.4, 21.787) -> (1.0507, 22.9312) centre (0.4, 22.1071) ccw projected
  line L2 (1.4, 21.787) -> (1.4, -1.787) projected
  arc A1 (1.0507, -2.9312) -> (1.4, -1.787) centre (0.4, -2.1071) ccw projected
  arc A2 (-7.0507, -2.9312) -> (1.0507, -2.9312) centre (-3, 0) ccw projected
  arc A3 (-7.4, -1.787) -> (-7.0507, -2.9312) centre (-6.4, -2.1071) ccw projected
  line L3 (-7.4, -1.787) -> (-7.4, 21.787) projected
  arc A4 (-7.0507, 22.9312) -> (-7.4, 21.787) centre (-6.4, 22.1071) ccw projected
  arc A5 (1.0507, 22.9312) -> (-7.0507, 22.9312) centre (-3, 20) ccw projected
  circle A6 centre (-6, -10) radius 1.35 projected
  circle A7 centre (0, -10) radius 1.35 projected
  circle A8 centre (-3, 40) radius 4 projected
  line L4 (9.45, -12) -> (9.45, 1.1169) projected
  arc A9 (9.45, 1.1169) -> (9.402, 1.5625) centre (-3, 0) ccw projected
  line L5 (4.4412, 40.9375) -> (9.402, 1.5625) projected
  arc A10 (4.4412, 40.9375) -> (-10.4412, 40.9375) centre (-3, 40) ccw projected
  line L6 (-10.4412, 40.9375) -> (-16.45, -6.7561) projected
  line L7 (-16.45, -6.7561) -> (-16.45, -12) projected
  line L8 (-16.45, -12) -> (9.45, -12) projected
  line L9 (-16.45, -8) -> (9.45, -8) projected
  line L10 (-16.45, -8) -> (-16.45, -12)
  line L11 (-16.45, -12) -> (-12.45, -12)
  line L12 (-12.45, -12) -> (-12.45, -8)
  line L13 (-12.45, -8) -> (-16.45, -8)
  line L14 (9.45, -8) -> (9.45, -12)
  line L15 (9.45, -12) -> (5.45, -12)
  line L16 (5.45, -12) -> (5.45, -8)
  line L17 (5.45, -8) -> (9.45, -8)
  line L18 (5.39, -7.94) -> (5.39, -12.06)
  line L19 (5.39, -12.06) -> (9.51, -12.06)
  line L20 (9.51, -12.06) -> (9.51, -7.94)
  line L21 (9.51, -7.94) -> (5.39, -7.94)
  line L22 (-12.39, -7.94) -> (-12.39, -12.06)
  line L23 (-12.39, -12.06) -> (-16.51, -12.06)
  line L24 (-16.51, -12.06) -> (-16.51, -7.94)
  line L25 (-16.51, -7.94) -> (-12.39, -7.94)
  point P0 (0, 0)
  dimension "d87" = 4
  dimension "d88" = 4
  dimension "d89" = 0.06
  dimension "d90" = 0.06
  constraints: 32 end point, 8 parallel, 6 perpendicular, 6 other
  measures "d87" distance of L11.end L7.end
  measures "d88" distance of L4.start L15.end
  measures "d89" distance between parallel lines of L16 L18
  measures "d90" distance between parallel lines of L12 L22
extrude "돌출24" cut sketch "스케치24" against normal blind 3 contours L4 L21 L20 L19 L18 L0 | L0 L16 L9 L4 | L0 L18 L9 L16 | L9 L18 L21 L4 | L22 L23 L24 L25 L7 L0 | L0 L12 L9 L22 | L0 L7 L9 L12 | L9 L7 L25 L22
sketch "스케치25" plane through (0, 0, 0) normal (0, 0, -1) x (-1, 0, 0)
  line L0 (5.39, -7.94) -> (9.45, -7.94) projected
  line L1 (9.45, -7.94) -> (9.45, 1.1169) projected
  arc A0 (9.45, 1.1169) -> (9.402, 1.5625) centre (-3, 0) ccw projected
  line L2 (4.4412, 40.9375) -> (9.402, 1.5625) projected
  arc A1 (4.4412, 40.9375) -> (-10.4412, 40.9375) centre (-3, 40) ccw projected
  line L3 (-10.4412, 40.9375) -> (-16.45, -6.7561) projected
  line L4 (-16.45, -6.7561) -> (-16.45, -7.94) projected
  line L5 (-16.45, -7.94) -> (-12.39, -7.94) projected
  line L6 (-12.39, -7.94) -> (-12.39, -12) projected
  line L7 (-12.39, -12) -> (5.39, -12) projected
  line L8 (5.39, -12) -> (5.39, -7.94) projected
  arc A2 (1.4, 21.787) -> (1.0507, 22.9312) centre (0.4, 22.1071) ccw projected
  line L9 (1.4, 21.787) -> (1.4, -1.787) projected
  arc A3 (1.0507, -2.9312) -> (1.4, -1.787) centre (0.4, -2.1071) ccw projected
  arc A4 (-7.0507, -2.9312) -> (1.0507, -2.9312) centre (-3, 0) ccw projected
  arc A5 (-7.4, -1.787) -> (-7.0507, -2.9312) centre (-6.4, -2.1071) ccw projected
  line L10 (-7.4, -1.787) -> (-7.4, 21.787) projected
  arc A6 (-7.0507, 22.9312) -> (-7.4, 21.787) centre (-6.4, 22.1071) ccw projected
  arc A7 (1.0507, 22.9312) -> (-7.0507, 22.9312) centre (-3, 20) ccw projected
  circle A8 centre (-6, -10) radius 1.35 projected
  circle A9 centre (0, -10) radius 1.35 projected
  circle A10 centre (-3, 40) radius 4 projected
  circle A11 centre (-12.39, -7.94) radius 1.1
  circle A12 centre (5.39, -7.94) radius 1.1
  point P0 (0, 0)
  dimension "d93" = 2.2
  dimension "d94" = 2.2
  constraints: 2 centre point, 2 coincident
  measures "d93" diameter of A11
  measures "d94" diameter of A12
extrude "돌출25" cut sketch "스케치25" against normal through all contours L8 A12 L0 | L0 A12 L8 | A11 L5 L6 | L6 L5 A11
sketch "스케치26" plane through (0, 0, 0) normal (0, 0, -1) x (-1, 0, 0)
  circle A0 centre (-3, 40) radius 4 projected
  circle A1 centre (0, -10) radius 1.35 projected
  circle A2 centre (-6, -10) radius 1.35 projected
  arc A3 (1.4, 21.787) -> (1.0507, 22.9312) centre (0.4, 22.1071) ccw projected
  line L0 (1.4, 21.787) -> (1.4, -1.787) projected
  arc A4 (1.0507, -2.9312) -> (1.4, -1.787) centre (0.4, -2.1071) ccw projected
  arc A5 (-7.0507, -2.9312) -> (1.0507, -2.9312) centre (-3, 0) ccw projected
  arc A6 (-7.4, -1.787) -> (-7.0507, -2.9312) centre (-6.4, -2.1071) ccw projected
  line L1 (-7.4, -1.787) -> (-7.4, 21.787) projected
  arc A7 (-7.0507, 22.9312) -> (-7.4, 21.787) centre (-6.4, 22.1071) ccw projected
  arc A8 (1.0507, 22.9312) -> (-7.0507, 22.9312) centre (-3, 20) ccw projected
  arc A9 (6.49, -7.94) -> (5.39, -9.04) centre (5.39, -7.94) ccw projected
  line L2 (6.49, -7.94) -> (9.45, -7.94) projected
  line L3 (9.45, -7.94) -> (9.45, 1.1169) projected
  arc A10 (9.45, 1.1169) -> (9.402, 1.5625) centre (-3, 0) ccw projected
  line L4 (4.4412, 40.9375) -> (9.402, 1.5625) projected
  arc A11 (4.4412, 40.9375) -> (-10.4412, 40.9375) centre (-3, 40) ccw projected
  line L5 (-10.4412, 40.9375) -> (-16.45, -6.7561) projected
  line L6 (-16.45, -6.7561) -> (-16.45, -7.94) projected
  line L7 (-16.45, -7.94) -> (-13.49, -7.94) projected
  arc A12 (-12.39, -9.04) -> (-13.49, -7.94) centre (-12.39, -7.94) ccw projected
  line L8 (-12.39, -9.04) -> (-12.39, -12) projected
  line L9 (-12.39, -12) -> (5.39, -12) projected
  line L10 (5.39, -12) -> (5.39, -9.04) projected
  line L11 (-16.45, -16.06) -> (9.45, -16.06)
  line L12 (9.45, -16.06) -> (9.45, -7.94)
  line L13 (9.45, -7.94) -> (-16.45, -7.94)
  line L14 (-16.45, -7.94) -> (-16.45, -16.06)
  line L15 (5.39, -12) -> (-12.39, -12) projected
  line L16 (-16.45, -16.06) -> (9.45, -7.94) construction
  line L17 (9.45, -16.06) -> (-16.45, -7.94) construction
  line L18 (-16.45, -7.94) -> (9.45, -7.94)
  line L19 (9.45, -7.94) -> (9.45, -3.94)
  line L20 (9.45, -3.94) -> (-16.45, -3.94)
  line L21 (-16.45, -3.94) -> (-16.45, -7.94)
  line L22 (-16.45, -3.94) -> (-9.8973, 45.001)
  point P0 (0, 0)
  point P1 (-3.5, -12)
  point P2 (-16.45, -6.7561)
  point P3 (-10.4337, 40.9953)
  dimension "d97" = 4
  constraints: 22 end point, 4 parallel, 3 midpoint, 3 perpendicular, 1 horizontal, 1 tangent
  measures "d97" distance of L19.end L2.end
extrude "돌출26" add sketch "스케치26" against normal up to surface (3 mm away) contours L20 L22 L5 | L5 L21 L20
sketch "스케치27" plane through (0, 0, 3) normal (0, 0, 1) x (1, 0, 0)
  arc A0 (-5.39, -9.04) -> (-6.49, -7.94) centre (-5.39, -7.94) ccw projected
  line L0 (-5.39, -9.04) -> (-5.39, -12) projected
  line L1 (-5.39, -12) -> (12.39, -12) projected
  line L2 (12.39, -12) -> (12.39, -9.04) projected
  arc A1 (13.49, -7.94) -> (12.39, -9.04) centre (12.39, -7.94) ccw projected
  line L3 (13.49, -7.94) -> (16.45, -7.94) projected
  line L4 (16.45, -7.94) -> (16.45, -3.94) projected
  line L5 (10.4337, 40.9953) -> (16.45, -3.94) projected
  arc A2 (10.4337, 40.9953) -> (-4.4412, 40.9375) centre (3, 40) ccw projected
  line L6 (-4.4412, 40.9375) -> (-9.402, 1.5625) projected
  arc A3 (-9.402, 1.5625) -> (-9.45, 1.1169) centre (3, 0) ccw projected
  line L7 (-9.45, 1.1169) -> (-9.45, -7.94) projected
  line L8 (-9.45, -7.94) -> (-6.49, -7.94) projected
  circle A4 centre (6, -10) radius 1.35 projected
  circle A5 centre (0, -10) radius 1.35 projected
  circle A6 centre (3, 40) radius 4 projected
  arc A7 (-1.0507, 22.9312) -> (-1.4, 21.787) centre (-0.4, 22.1071) ccw projected
  arc A8 (7.0507, 22.9312) -> (-1.0507, 22.9312) centre (3, 20) ccw projected
  arc A9 (7.4, 21.787) -> (7.0507, 22.9312) centre (6.4, 22.1071) ccw projected
  line L9 (7.4, 21.787) -> (7.4, -1.787) projected
  arc A10 (7.0507, -2.9312) -> (7.4, -1.787) centre (6.4, -2.1071) ccw projected
  arc A11 (-1.0507, -2.9312) -> (7.0507, -2.9312) centre (3, 0) ccw projected
  arc A12 (-1.4, -1.787) -> (-1.0507, -2.9312) centre (-0.4, -2.1071) ccw projected
  line L10 (-1.4, -1.787) -> (-1.4, 21.787) projected
  line L11 (16.45, -7.94) -> (16.45, -3.94)
  line L12 (16.45, -3.94) -> (-9.45, -3.94)
  line L13 (-9.45, -3.94) -> (-9.45, -7.94)
  line L14 (-9.45, -7.94) -> (16.45, -7.94)
  line L15 (-9.45, -3.94) -> (-3.7438, 47.1935)
  arc A13 (10.4337, 40.9953) -> (-4.4412, 40.9375) centre (3, 40) ccw projected
  point P0 (0, 0)
  point P1 (-9.45, -3.94)
  point P2 (-4.4478, 40.8847)
  constraints: 10 end point, 2 parallel, 1 perpendicular, 1 tangent, 1 vertical
extrude "돌출27" cut sketch "스케치27" against normal through all contours L7 A3 L6 L15
